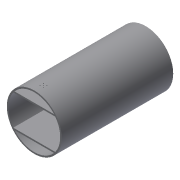
# Autodesk Inventor part: Chassis
Saved by Autodesk Inventor 2017 (Build 210142000, 142)
## iProperties
Created: 2017-03-13
Part Number: Chassis
Material: Generic
Document SubType Name: Modeling
Designer: zallen
Density: 1 g/cm^3
Appearance: Default
Author: zallen
Autodesk Inventor part; units mm, degrees
ref_plane "YZ Plane" through (0, 0, 0) normal (1, 0, 0) x (0, 1, 0)
ref_plane "XZ Plane" through (0, 0, 0) normal (0, 1, 0) x (-1, 0, 0)
ref_plane "XY Plane" through (0, 0, 0) normal (0, 0, 1) x (1, 0, 0)
sketch "Sketch1" plane through (0, 0, 0) normal (0, 0, 1) x (1, 0, 0)
  circle A0 centre (0, 0) radius 228.6
  dimension "d0" = 457.2
  constraints: 1 centre point, 1 coincident
  measures "d0" diameter of A0
extrude "Extrusion1" add sketch "Sketch1" along normal blind 12.7
sketch "Sketch2" plane through (0, 0, 12.7) normal (0, 0, 1) x (1, 0, 0)
  circle A0 centre (0, 0) radius 228.6
  circle A1 centre (0, 0) radius 215.9
  dimension "d3" = 457.2
  dimension "d4" = 431.8
  constraints: 2 centre point, 2 coincident
  measures "d3" diameter of A0
  measures "d4" diameter of A1
extrude "Extrusion2" add sketch "Sketch2" along normal blind 914.4
sketch "Sketch3" plane through (0, 0, 12.7) normal (0, 0, 1) x (1, 0, 0)
  line L0 (0, -139.7) -> (164.6108, -139.7)
  line L1 (0, -127) -> (174.5961, -127)
  circle A0 centre (0, 0) radius 215.9 projected
  circle A1 centre (0, 0) radius 215.9 projected
  line L2 (0, 127) -> (174.5961, 127)
  line L3 (0, 139.7) -> (164.6108, 139.7)
  line L4 (0, 139.7) -> (-164.6108, 139.7)
  line L5 (0, 127) -> (-174.5961, 127)
  circle A2 centre (0, 0) radius 215.9
  line L6 (0, -127) -> (-174.5961, -127)
  line L7 (0, -139.7) -> (-164.6108, -139.7)
  dimension "d7" = 12.7
  dimension "d8" = 127
  dimension "d9" = 12.7
  dimension "d10" = 127
  constraints: 16 end point, 8 horizontal, 1 centre point, 1 coincident, 9 other
  measures "d7" distance of L1.start L0.start
  measures "d8" distance of point (0, 0) L1.start
  measures "d9" distance of L3.start L2.start
  measures "d10" distance of point (0, 0) L2.start
extrude "Extrusion3" add sketch "Sketch3" along normal blind 914.4 contours L7 A0 L6 L1 L0 | A0 L4 L3 L2 L5
sketch "Sketch4" plane through (-164.6108, 139.7, 12.7) normal (0, 1, 0) x (1, 0, 0)
  circle A0 centre (179.3705, -852.342) radius 3.175
  circle A1 centre (151.0865, -852.342) radius 3.175
  circle A2 centre (179.3705, -824.058) radius 3.175
  circle A3 centre (151.0749, -824.058) radius 3.175
  circle A4 centre (165.2169, -838.2) radius 3.175
  line L0 (-63.9892, -914.4) -> (393.2108, -914.4) projected
  line L1 (339.2069, -914.4) -> (339.2069, 0) projected
  point P0 (164.6108, 12.7)
  dimension "d13" = 6.35
  dimension "d14" = 6.35
  dimension "d15" = 6.35
  dimension "d16" = 6.35
  dimension "d17" = 28.284
  dimension "d18" = 28.284
  dimension "d19" = 28.2956
  dimension "d20" = 28.284
  dimension "d21" = 28.284
  dimension "d22" = 28.284
  dimension "d23" = 6.35
  dimension "d24" = 14.142
  dimension "d25" = 14.142
  dimension "d26" = 76.2
  dimension "d27" = 173.99
  constraints: 5 centre point
  measures "d13" diameter of A0
  measures "d14" diameter of A1
  measures "d15" diameter of A2
  measures "d16" diameter of A3
  measures "d17" distance of A1.centre A0.centre
  measures "d18" distance of A2.centre A0.centre
  measures "d19" distance of A3.centre A2.centre
  measures "d20" distance of A1.centre A3.centre
  measures "d21" vertical distance of A3.centre A0.centre
  measures "d22" horizontal distance of A1.centre A2.centre
  measures "d23" diameter of A4
  measures "d24" vertical distance of A4.centre A0.centre
  measures "d25" horizontal distance of A3.centre A4.centre
  measures "d26" distance from line of L0 A4.centre
  measures "d27" distance from line of L1 A4.centre
extrude "Extrusion4" cut sketch "Sketch4" along normal blind 914.4
body "Solid1"
